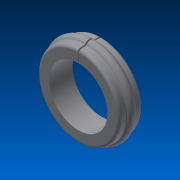
# Autodesk Inventor part: anel rotacao sonda completo com gap
Saved by Autodesk Inventor 2015 (Build 190159000, 159)
## iProperties
Created: 2015-12-29
Part Number: anel rotacao sonda completo com gap
Material: Genérico
Document SubType Name: Modeling
Designer: hp
Density: 1 g/cm^3
Appearance: Padrão
Author: hp
Autodesk Inventor part; units mm, degrees
ref_plane "YZ Plane" through (0, 0, 0) normal (1, 0, 0) x (0, 1, 0)
ref_plane "XZ Plane" through (0, 0, 0) normal (0, 1, 0) x (-1, 0, 0)
ref_plane "XY Plane" through (0, 0, 0) normal (0, 0, 1) x (1, 0, 0)
sketch "Esboço1" plane through (0, 0, 0) normal (0, 1, 0) x (-1, 0, 0)
  circle A0 centre (0, 0) radius 15
  circle A1 centre (0, 0) radius 9.95
  dimension "d0" = 30
  dimension "d1" = 19.9
  constraints: 2 centre point, 2 coincident
  measures "d0" diameter of A0
  measures "d1" diameter of A1
extrude "Extrusão1" add sketch "Esboço1" along normal blind 8
sketch "Esboço2" plane through (0, 8, 0) normal (0, 1, 0) x (1, 0, 0)
  circle A0 centre (0, 0) radius 15
  circle A1 centre (0, 0) radius 14
  dimension "d4" = 30
  dimension "d5" = 28
  constraints: 2 centre point, 2 coincident
  measures "d4" diameter of A0
  measures "d5" diameter of A1
extrude "Extrusão2" cut sketch "Esboço2" against normal blind 2.5
sketch "Esboço3" plane through (0, 0, 0) normal (0, -1, 0) x (1, 0, 0)
  circle A0 centre (0, 0) radius 15
  circle A1 centre (0, 0) radius 14 projected
  circle A2 centre (0, 0) radius 14
  dimension "d8" = 30
  constraints: 2 centre point, 2 coincident
  measures "d8" diameter of A0
extrude "Extrusão3" cut sketch "Esboço3" against normal blind 2.5
fillet "Arredondamento1" radius 1.5 1 edges at (15, 2.5, 0)
fillet "Arredondamento2" radius 1.5 1 edges at (15, 5.5, 0)
fillet "Arredondamento3" radius 1 2 edges at (-14, 0, 0) (-14, 8, 0)
fillet "Arredondamento4" radius 0.5 4 edges at (0, 2.5, 14) (0, 2.5, -14) (0, 5.5, 14) (0, 5.5, -14)
sketch "Esboço4" plane through (0, 0, 0) normal (0, -1, 0) x (1, 0, 0)
  line L0 (0, 0) -> (-0.3141, 17.9973)
  line L1 (0, 0) -> (18, 0) construction
  line L2 (0, 0) -> (0.3141, 17.9973)
  line L3 (0, 0) -> (18, 0) construction
  line L4 (0.3141, 17.9973) -> (-0.3141, 17.9973)
  dimension "d15" = 18
  dimension "d16" = 91
  dimension "d17" = 18
  dimension "d18" = 89
  constraints: 10 end point, 2 equal length, 2 horizontal
  measures "d15" distance of L0.start L0.end
  measures "d16" angle of L1 L0
  measures "d17" distance of L0.start L2.end
  measures "d18" angle of L3 L2
extrude "Extrusão4" cut sketch "Esboço4" against normal up to surface (8 mm away)
